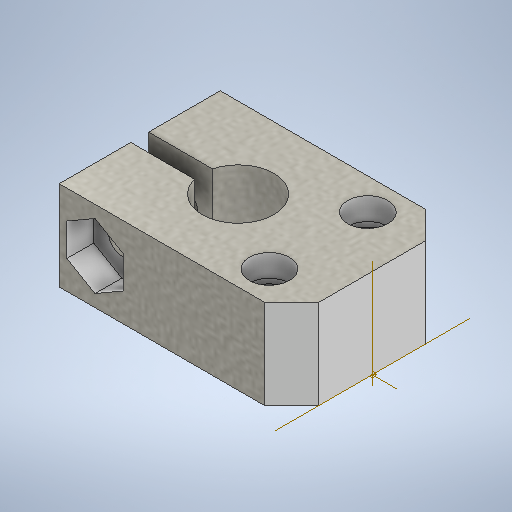
# Autodesk Inventor part: Shaft support
Saved by Autodesk Inventor 2025.2 (Build 292293000, 293)
## iProperties
Created: 2025-01-25
Part Number: Shaft support
Material: Generic
Document SubType Name: Modeling
Designer: caomi
Density: 1 g/cm^3
Appearance: Default
Author: caomi
Autodesk Inventor part; units mm, degrees
ref_plane "YZ Plane" through (0, 0, 0) normal (1, 0, 0) x (0, 1, 0)
ref_plane "XZ Plane" through (0, 0, 0) normal (0, 1, 0) x (-1, 0, 0)
ref_plane "XY Plane" through (0, 0, 0) normal (0, 0, 1) x (1, 0, 0)
sketch "Sketch1" plane through (0, 0, 0) normal (0, 1, 0) x (-1, 0, 0)
  line L0 (11, 0) -> (0, 0)
  line L1 (0, -9) -> (26, -9)
  line L2 (26, -9) -> (26, -1)
  circle A0 centre (15, 0) radius 4
  line L3 (18.873, -1) -> (26, -1)
  line L4 (0, 9) -> (26, 9)
  line L5 (26, 9) -> (26, 1)
  circle A1 centre (15, 0) radius 4
  line L6 (18.873, 1) -> (26, 1)
  line L7 (0, -9) -> (0, 0)
  line L8 (0, 9) -> (0, 0)
  point P0 (18.873, 1)
  dimension "d2" = 1
  dimension "d3" = 9
  dimension "d4" = 8
  dimension "d27" = 15
  dimension "d28" = 26
  constraints: 18 end point, 4 symmetric about line, 2 horizontal, 2 point on circle, 2 point on line, 1 centre point, 1 line through centre, 1 perpendicular, 1 vertical, 3 other
  measures "d2" distance between parallel lines of L3 L0
  measures "d3" distance between parallel lines of L1 L0
  measures "d4" diameter of A0
  measures "d27" distance from line of L7 A0.centre
  measures "d28" distance between parallel lines of L7 L2
extrude "Extrusion1" add sketch "Sketch1" along normal blind 10 contours A0 L3 L2 L1 L7 L0 | L0 L8 L4 L5 L6 A0
sketch "Sketch7" plane through (0, 10, 0) normal (0, 1, 0) x (1, 0, 0)
  line L0 (0, -9) -> (0, 9) projected
  line L1 (-31.2, 0) -> (5.2, 0) projected
  point P0 (0, 0)
  point P1 (-6, -5.5)
  point P2 (0, 0)
  point P3 (-6, 5.5)
  dimension "d33" = 6
  dimension "d44" = 11
  constraints: 1 midpoint, 1 symmetric about line, 1 vertical alignment
  measures "d33" distance from line of point (-6, -5.5) L0
  measures "d44" distance of point (-6, 5.5) point (-6, -5.5)
hole "Hole1" at (-6, 10, 5.5) at (-6, 10, -5.5) direction (0, -1, 0) diameter 3 end through all counterbore diameter 4.5 counterbore depth 2.5
sketch "Sketch3" plane through (0, 0, -9) normal (0, 0, -1) x (-1, 0, 0)
  circle A0 centre (22, 5) radius 1.5
  line L0 (26, 0) -> (26, 10) projected
  point P0 (0, 0)
  point P1 (26, 5)
  dimension "d15" = 3
  dimension "d16" = 4
  constraints: 1 centre point, 1 horizontal alignment, 1 midpoint
  measures "d15" diameter of A0
  measures "d16" distance from line of A0.centre L0
extrude "Extrusion3" cut sketch "Sketch3" against normal up to surface (18 mm away)
sketch "Sketch4" plane through (-26, 0, 9) normal (0, 0, 1) x (1, 0, 0)
  line L0 (0.85, 6.8187) -> (4, 8.6373)
  line L1 (4, 8.6373) -> (7.15, 6.8187)
  line L2 (7.15, 6.8187) -> (7.15, 3.1813)
  line L3 (7.15, 3.1813) -> (4, 1.3627)
  line L4 (4, 1.3627) -> (0.85, 3.1813)
  line L5 (0.85, 3.1813) -> (0.85, 6.8187)
  circle A0 centre (4, 5) radius 1.5 projected
  point P0 (26, 0)
  point P1 (0.85, 5)
  dimension "d20" = 6.3
  constraints: 12 end point, 1 coincident, 1 midpoint, 1 vertical, 13 other
  measures "d20" distance from line of L2 point (0.85, 5)
extrude "Extrusion4" cut sketch "Sketch4" against normal blind 3
sketch "Sketch5" plane through (0, 0, -9) normal (0, 0, -1) x (-1, 0, 0)
  circle A0 centre (22, 5) radius 2.35
  circle A1 centre (22, 5) radius 1.5 projected
  point P0 (0, 0)
  dimension "d23" = 4.7
  constraints: 1 centre point, 1 coincident
  measures "d23" diameter of A0
extrude "Extrusion5" cut sketch "Sketch5" against normal blind 2 contours A0 | A1
chamfer "Chamfer1" distance 3 angle 45 2 edges at (0, 5, 9) (0, 5, -9)
equation "\"d17\" = d15"
body "Solid1"
